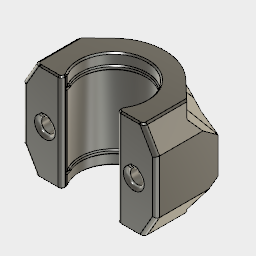
y_bearing_holder (Autodesk Fusion 360 design; units mm, degrees)
Autodesk Fusion 360 part; units mm, degrees
sketch "base" plane through (0, 0, 0) normal (0, 0, 1) x (1, 0, 0)
  circle A0 centre (0, 0) radius 7.525
  line L0 (-15, -5.4) -> (15, -5.4)
  line L1 (15, -5.4) -> (15, 1.6)
  line L2 (15, 1.6) -> (7.9667, 8.3281)
  line L3 (-15, -5.4) -> (-15, 1.6)
  line L4 (-15, 1.6) -> (-7.9667, 8.3281)
  line L5 (0, 54) -> (0, -54) construction
  arc A1 (7.9667, 8.3281) -> (-7.9667, 8.3281) centre (0, 0) ccw
  circle A2 centre (0, 0) radius 7.275
  line L6 (-6.25, -3.7233) -> (-6.25, -5.4)
  line L7 (6.25, -3.7233) -> (6.25, -5.4)
  line L8 (-24.9981, -5.711) -> (-4.9, -5.711) construction
  line L9 (-4.9, -5.711) -> (-4.9, -11.711) construction
  line L10 (-4.9, -11.711) -> (-24.9981, -11.711) construction
  line L11 (-24.9981, -11.711) -> (-24.9981, -5.711) construction
  line L12 (15, 1.6) -> (15, 8.6)
  line L13 (15, 8.6) -> (0, 8.6)
  line L14 (-15, 1.6) -> (-15, 8.6)
  line L15 (-15, 8.6) -> (0, 8.6)
  dimension "d1" = 15.05
  dimension "d3" = 7
  dimension "d8" = 4
  dimension "d11" = 12.5
  dimension "d88" = 4.9
  dimension "d90" = 6
  dimension "d115" = 5.4
  dimension "d117" = 0.311
  dimension "d118" = 15
  dimension "d126" = 0.25
  dimension "d162" = 14
  measures "d1" diameter of A0
  measures "d3" distance of L0.end L1.end
  measures "d8" distance of A0 A1
  measures "d11" distance of L6.end L7.end
  measures "d88" distance of L5 L9
  measures "d90" distance of L8.start L10.end
  measures "d115" distance of L0 A0.centre
  measures "d117" distance of L0 L8
  measures "d118" distance of L0.end A0.centre
  measures "d126" distance of A0 A2
  measures "d162" distance of L0.end L12.end
extrude "Extrude1" add sketch "base" along normal blind 16.4 contours A0 L0 L1 L2 L3 L4 A1 L6 L7 L13 L15 | A1 L13 L15
extrude "Extrude2" add sketch "base" along normal mid plane 1 contours A0 A2 L6 L7 | A0 L0 L1 L2 L3 L4 A1 L6 L7 L13 L15 | A1 L13 L15
extrude "Extrude3" add sketch "base" along normal mid plane 1 from surface at 16.4 contours A0 A2 L6 L7 | A0 L0 L1 L2 L3 L4 A1 L6 L7 L13 L15 | A1 L13 L15
extrude "Extrude9" add sketch "base" against normal blind 2.8 contours A0 L0 L1 L2 L3 L4 A1 L6 L7 L13 L15 | A1 L13 L15
extrude "Extrude10" add sketch "base" along normal blind 2.3 from surface at 16.9 contours A0 L0 L1 L2 L3 L4 A1 L6 L7 L13 L15 | A1 L13 L15
extrude "Extrude15" add sketch "base" along normal mid plane 8 from surface at 7.7 contours L4 A1 L14 L15 | L2 A1 L12 L13
chamfer "Chamfer11" distance 3.5 angle 45 2 edges at (-7.6724, 8.6, 7.7) (7.6724, 8.6, 7.7)
sketch "screw_holes" plane through (0, -5.4, 0) normal (0, -1, 0) x (1, 0, 0)
  line L0 (-15, 19.2) -> (-15, -2.8)
  line L1 (-15, -2.8) -> (-15, 19.2)
  circle A0 centre (-10, 7.7) radius 1.325
  circle A1 centre (10, 7.7) radius 1.325
  line L2 (10, 7.7) -> (-10, 7.7) construction
  line L3 (0, 0) -> (0, 23.025) construction
  line L4 (-10.6625, 8.8475) -> (-10.334, 9.176)
  line L5 (-10.334, 9.176) -> (-9.666, 9.176)
  line L6 (-9.666, 9.176) -> (-9.3375, 8.8475)
  line L7 (-10, 7.7) -> (-10, 9.176) construction
  line L8 (-15, 2.2) -> (-12.1132, -2.8)
  line L9 (-15, 14.2) -> (-12.1132, 19.2)
  line L10 (12.1132, 19.2) -> (15, 14.2)
  line L11 (15, 2.2) -> (12.1132, -2.8)
  circle A2 centre (-10, 7.7) radius 1.55
  line L12 (-10.775, 9.0423) -> (-10.4163, 9.401)
  line L13 (-10.4163, 9.401) -> (-9.5837, 9.401)
  line L14 (-9.5837, 9.401) -> (-9.225, 9.0423)
  line L15 (-10, 9.176) -> (-10, 9.401) construction
  circle A3 centre (10, 7.7) radius 1.55
  line L16 (10.4163, 9.401) -> (9.5837, 9.401)
  line L17 (9.5837, 9.401) -> (9.225, 9.0423)
  line L18 (10.775, 9.0423) -> (10.4163, 9.401)
  line L19 (10.334, 9.176) -> (9.666, 9.176)
  line L20 (9.666, 9.176) -> (9.3375, 8.8475)
  line L21 (10.6625, 8.8475) -> (10.334, 9.176)
  line L22 (-6.25, 19.2) -> (-15, 19.2)
  line L23 (-15, -2.8) -> (-6.25, -2.8)
  line L24 (15, -2.8) -> (6.25, -2.8)
  line L25 (6.25, 19.2) -> (15, 19.2)
  circle A4 centre (-10, 7.7) radius 2.775 construction
  line L26 (-12.775, 6.0979) -> (-10, 4.4957)
  line L27 (-10, 4.4957) -> (-7.225, 6.0979)
  line L28 (-7.225, 6.0979) -> (-7.225, 9.3021)
  line L29 (-7.225, 9.3021) -> (-10, 10.9043)
  line L30 (-10, 10.9043) -> (-12.775, 9.3021)
  line L31 (-12.775, 9.3021) -> (-12.775, 6.0979)
  line L32 (12.775, 6.0979) -> (10, 4.4957)
  line L33 (10, 4.4957) -> (7.225, 6.0979)
  line L34 (7.225, 6.0979) -> (7.225, 9.3021)
  line L35 (7.225, 9.3021) -> (10, 10.9043)
  line L36 (12.775, 9.3021) -> (12.775, 6.0979)
  line L37 (10, 10.9043) -> (12.775, 9.3021)
  line L38 (15, 11.7) -> (15, 19.2)
  line L39 (15, -2.8) -> (15, 3.7)
  point P0 (-10, 7.7)
  dimension "d19" = 2.65
  dimension "d20" = 10.5
  dimension "d23" = 20
  dimension "d32" = 0.151
  dimension "d39" = 1.325
  dimension "d43" = 45
  dimension "d44" = 45
  dimension "d54" = 5
  dimension "d72" = 3.1
  dimension "d73" = 0.151
  dimension "d74" = 45
  dimension "d75" = 1.55
  dimension "d130" = 60
  dimension "d131" = 60
  dimension "d132" = 60
  dimension "d133" = 60
  dimension "d135" = 5
  dimension "d151" = 5.55
  dimension "d159" = 5
  dimension "d160" = 5
  measures "d19" diameter of A0
  measures "d20" distance of L0.end P0
  measures "d23" distance of P0 A1.centre
  measures "d32" distance of A0 L5
  measures "d39" distance of L4.start L6.end
  measures "d43" angle of L4 L5
  measures "d44" angle of L5 L6
  measures "d54" distance of L0.start L9.start
  measures "d72" diameter of A2
  measures "d73" distance of A2 L13
  measures "d74" angle of L12 L13
  measures "d75" distance of L12.start L14.end
  measures "d130" angle of L9 L22
  measures "d131" angle of L10 L25
  measures "d132" angle of L8 L23
  measures "d133" angle of L11 L24
  measures "d135" distance of L0.end L8.start
  measures "d151" diameter of A4
  measures "d159" distance of L10.end L25.end
  measures "d160" distance of L11.start L24.start
extrude "Extrude4" cut sketch "screw_holes" against normal blind 25 contours L0 L1 L9 L22 | L0 L1 L8 L23 | L10 L25 L38 | L11 L24 L39
extrude "Extrude6" cut sketch "screw_holes" against normal blind 22 contours A0 | A0 L4 L5 L6 | A1 | A1 L19 L20 L21 | A2 | A2 L12 L13 L14 | A3 | A3 L16 L17 L18
extrude "Extrude14" cut sketch "screw_holes" against normal blind 9 from surface at -11.5 contours L26 L27 L28 L29 L30 L31 | L32 L33 L34 L35 L36 L37
chamfer "Chamfer9" distance 5.058 angle 45 8 edges at (11.4834, 4.964, 11.7) (6.4446, 9.5547, 11.7) (-6.4446, 9.5547, 3.7) (6.4446, 9.5547, 3.7) (11.4834, 4.964, 3.7) (-11.4834, 4.964, 3.7) (-6.4446, 9.5547, 11.7) (-11.4834, 4.964, 11.7)
sketch "bearing_fillets" plane through (0, 0, -2.8) normal (0, 0, -1) x (1, 0, 0)
  line L0 (-12.1132, 5.4) -> (-12.1132, -4.3615)
  line L1 (-12.1132, -4.3615) -> (-7.9667, -8.3281)
  arc A0 (-7.9667, -8.3281) -> (7.9667, -8.3281) centre (0, 0) ccw
  line L2 (7.9667, -8.3281) -> (12.1132, -4.3615)
  line L3 (12.1132, -4.3615) -> (12.1132, 5.4)
  line L4 (12.1132, 5.4) -> (6.25, 5.4)
  line L5 (6.25, 5.4) -> (6.25, 4.1908)
  arc A1 (-6.25, 4.1908) -> (6.25, 4.1908) centre (0, 0) ccw
  line L6 (-6.25, 4.1908) -> (-6.25, 5.4)
  line L7 (-6.25, 5.4) -> (-12.1132, 5.4)
  line L8 (-6.25, 4.1908) -> (-6.25, 5.4)
  line L9 (-6.25, 5.4) -> (-12.1132, 5.4)
  line L10 (12.1132, 5.4) -> (6.25, 5.4)
  line L11 (6.25, 5.4) -> (6.25, 4.1908)
  arc A2 (-6.25, 4.1908) -> (6.25, 4.1908) centre (0, 0) ccw
  arc A3 (-6.25, 3.7233) -> (6.25, 3.7233) centre (0, 0) ccw
  line L12 (-6.25, 3.7233) -> (-6.25, 4.1908)
  line L13 (6.25, 4.1908) -> (6.25, 3.7233)
  line L14 (0, 0) -> (0, 5.4) construction
  arc A4 (-6.25, 4.6) -> (-7.049, 5.4) centre (-7.05, 4.6) ccw
  arc A5 (-6.3725, 4.0021) -> (-6.25, 4.4275) centre (-7.05, 4.4275) ccw
  arc A6 (-6.5349, 3.1971) -> (-6.25, 4.4275) centre (-9.05, 4.4275) ccw
  arc A7 (6.25, 4.4275) -> (6.5349, 3.1971) centre (9.05, 4.4275) ccw
  arc A8 (7.049, 5.4) -> (6.25, 4.6) centre (7.05, 4.6) ccw
  arc A9 (6.25, 4.4275) -> (6.3725, 4.0021) centre (7.05, 4.4275) ccw
  dimension "d177" = 0.8
  dimension "d178" = 0.8
  measures "d177" radius of A4
  measures "d178" radius of A5
extrude "Extrude11" cut sketch "bearing_fillets" against normal blind 25.5 contours L6 L7 L8 L9 A4 | A1 A2 A5 A6 | A1 L6 L8 A2 A6 | A1 A2 A3 L12 A6 | A1 A2 A7 A9 | L4 L5 L10 L11 A8 | A1 A2 A3 L13 A7 | L5 A1 L11 A2 A7
extrude "Extrude12" add sketch "bearing_fillets" against normal up to surface (1 mm away) from surface at -2.3 contours A1 A2 A5 A6 | A1 A2 A7 A9
extrude "Extrude13" add sketch "bearing_fillets" against normal up to surface (1 mm away) from surface at -18.7 contours A1 A2 A5 A6 | A1 A2 A7 A9
chamfer "Chamfer8" distance 0.25 angle 45 12 edges at (0, 7.275, -0.5) (0, 7.275, 0.5) (0, 7.275, 15.9) (0, 7.275, 16.9) (-6.3221, -3.796, -0.5) (-6.3221, -3.796, 0.5) (-6.3221, -3.796, 15.9) (-6.3221, -3.796, 16.9) (6.3221, -3.796, -0.5) (6.3221, -3.796, 0.5) (6.3221, -3.796, 15.9) (6.3221, -3.796, 16.9) tangent chain off
fillet "Fillet1" radius 0.8 6 edges at (-13.5566, -5.4, -0.3) (-15, -5.4, 8.2) (-13.5566, -5.4, 16.7) (13.5566, -5.4, 16.7) (15, -5.4, 8.2) (13.5566, -5.4, -0.3)
chamfer "Chamfer5" distance 0.3 angle 45 26 edges at (-9.1192, -5.4, -2.8) (-11.8427, -5.1657, -2.8) (-12.1132, -0.1193, -2.8) (0, 7.525, -2.8) (12.1132, -0.1193, -2.8) (11.8427, -5.1657, -2.8) (9.1192, -5.4, -2.8) (0, 7.525, 19.2) (9.1192, -5.4, 19.2) (11.8427, -5.1657, 19.2) (12.1132, -0.1193, 19.2) (-12.1132, -0.1193, 19.2) (-11.8427, -5.1657, 19.2) (-9.1192, -5.4, 19.2) (6.4839, -5.1653, 19.2) (6.2812, -4.2062, 19.2) (6.25, -4.5138, 19.2) (-6.2812, -4.2062, 19.2) (-6.25, -4.5138, 19.2) (-6.4839, -5.1653, 19.2) (-6.4839, -5.1653, -2.8) (-6.25, -4.5138, -2.8) (-6.2812, -4.2062, -2.8) (6.4839, -5.1653, -2.8) (6.25, -4.5138, -2.8) (6.2812, -4.2062, -2.8) tangent chain off
fillet "Fillet2" radius 0.8 8 edges at (-10, -5.4, 6.15) (-10.5957, -5.4, 9.2217) (-10, -5.4, 9.401) (-9.4043, -5.4, 9.2217) (10, -5.4, 6.15) (10, -5.4, 9.401) (9.4043, -5.4, 9.2217) (10.5957, -5.4, 9.2217)
extrude "Extrude16" cut 2 faces at (12.3667, 6.1, 7.7) (-11.1833, 6.1, 5.6504) along direction (0, 1, 0) blind 3 draft 10 from surface at 1.5
sketch "mk_type" plane through (-10.2974, 0, -5.9452) normal (-0.866025, 0, -0.5) x (0, -1, 0)
  line L0 (-4.218, 3.9318) -> (4.6, 3.9318)
  line L1 (4.6, 3.9318) -> (4.6, 9.4053)
  line L2 (4.6, 9.4053) -> (-6.5238, 9.4053)
  line L3 (-6.5238, 9.4053) -> (-3.5651, 5.2968)
  line L4 (-3.5651, 5.2968) -> (-4.218, 3.9318)
  line L5 (4.6, 9.4053) -> (4.6, 3.9318)
  line L6 (-3.5651, 5.2968) -> (-6.5238, 9.4053)
  line L7 (4.6, 6.6685) -> (-4.5529, 6.6685) construction
  circle A0 centre (-0.9765, 6.6685) radius 0.75
  circle A1 centre (1.0235, 6.6685) radius 0.75
  point P0 (0.0235, 6.6685)
  dimension "d180" = 1.5
  dimension "d181" = 1.5
  dimension "d182" = 1
  dimension "d183" = 1
  measures "d180" diameter of A0
  measures "d181" diameter of A1
  measures "d182" distance of A0.centre P0
  measures "d183" distance of A1.centre P0
extrude "Extrude17" cut sketch "mk_type" against normal blind 0.5 contours A0 | A1
equation "d1 = bearing_out_dia"
equation "d9 = groove_space"
equation "d12 = groove_width"
equation "d15 = -groove_width"
equation "d19 = m3_thread"
equation "d20 = bearing_length / 2 - 0.5 mm"
equation "d32 = layer_height + 0.001 mm"
equation "d39 = d19 / 2"
equation "num_perimeters = 4"
equation "extrusion_width = 0.45 mm"
equation "layer_height = 0.15 mm"
equation "perimeters_thickness = num_perimeters * extrusion_width - 0.1 mm"
equation "num_top_bottom = 5"
equation "top_bottom_thickness = num_top_bottom * layer_height"
equation "d72 = m3_hole"
equation "d73 = layer_height + 0.001 mm"
equation "d75 = d72 / 2"
equation "groove_space = 17.5 mm - 1.1 mm"
equation "bearing_out_dia = 15.0 mm + 0.05 mm"
equation "groove_depth = 0.35 mm - 0.10 mm"
equation "groove_width = 1.1 mm - 0.10 mm"
equation "d119 = -( bearing_length - groove_space ) / 2"
equation "d122 = ( bearing_length - groove_space - groove_width ) / 2"
equation "d126 = groove_depth"
equation "bearing_length = 24 mm - 2 mm"
equation "d131 = d130"
equation "d132 = d130"
equation "d133 = d130"
equation "d135 = d54"
equation "m3_thread = 2.65 mm"
equation "d146 = groove_depth"
equation "m3_hole = 3.1 mm"
equation "d151 = m3_nut_width"
equation "d152 = -nut_height"
equation "d156 = -bearing_length / 2 + 0.5 mm"
equation "d159 = d54"
equation "d160 = d54"
equation "nut_height = 11.5 mm"
equation "d162 = nut_height + 2.5 mm"
equation "m3_nut_width = 5.4 mm + 0.15 mm"
equation "d178 = d177"
equation "d181 = d180"
equation "d183 = d182"
